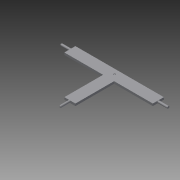
# Autodesk Inventor part: Motor_Mount
Saved by Autodesk Inventor 2015 (Build 190159000, 159)
## iProperties
Created: 2016-02-14
Part Number: Motor_Mount
Material: Generic
Document SubType Name: Modeling
Designer: david_000
Density: 1 g/cm^3
Appearance: Default
Author: david_000
Autodesk Inventor part; units mm, degrees
ref_plane "YZ Plane" through (0, 0, 0) normal (1, 0, 0) x (0, 1, 0)
ref_plane "XZ Plane" through (0, 0, 0) normal (0, 1, 0) x (-1, 0, 0)
ref_plane "XY Plane" through (0, 0, 0) normal (0, 0, 1) x (1, 0, 0)
sketch "Sketch1" plane through (0, 0, 0) normal (0, 1, 0) x (-1, 0, 0)
  line L0 (-254, 0) -> (-254, -31.75)
  line L1 (-254, -31.75) -> (0, -31.75)
  line L2 (0, -31.75) -> (0, 0)
  line L3 (-111.125, -15.875) -> (-142.875, -15.875)
  line L4 (-142.875, 0) -> (-142.875, 111.125)
  line L5 (-142.875, 111.125) -> (-111.125, 111.125)
  line L6 (-111.125, 111.125) -> (-111.125, 0)
  line L7 (0, 0) -> (-111.125, 0)
  line L8 (-142.875, 0) -> (-254, 0)
  point P0 (-127, -15.875)
  dimension "d0" = 254
  dimension "d1" = 31.75
  dimension "d5" = 15.875
  dimension "d6" = 127
  dimension "d7" = 15.875
  dimension "d8" = 127
  constraints: 18 end point, 5 parallel, 3 horizontal, 3 perpendicular
  measures "d0" distance of L1.end L0.end
  measures "d1" distance of L0.end L0.start
  measures "d5" distance of point (-127, -15.875) L3.start
  measures "d6" distance from line of L2 point (-127, -15.875)
  measures "d7" distance of point (-127, -15.875) point (-142.875, -15.875)
  measures "d8" distance of L3.end L4.end
extrude "Extrusion1" add sketch "Sketch1" along normal blind 6.35
sketch "Sketch3" plane through (0, 6.35, 0) normal (0, 1, 0) x (1, 0, 0)
  line L0 (0, 0) -> (111.125, 0) projected
  line L1 (0, 31.75) -> (0, 0) projected
  circle A0 centre (127, 17.145) radius 3.3156
  dimension "d13" = 17.145
  dimension "d14" = 127
  constraints: 1 centre point, 1 coincident
  measures "d13" distance from line of L0 point (127, 17.145)
  measures "d14" distance from line of L1 point (127, 17.145)
extrude "Extrusion3" cut sketch "Sketch3" against normal blind 1.27
sketch "Sketch4" plane through (254, 0, 0) normal (1, 0, 0) x (0, 0, -1)
  line L0 (31.75, 0) -> (0, 0) projected
  line L1 (31.75, 0) -> (31.75, 6.35) projected
  circle A0 centre (15.875, 3.175) radius 3.175
  dimension "d21" = 15.875
  dimension "d22" = 3.175
  constraints: 1 centre point, 1 coincident
  measures "d21" distance from line of L1 point (15.875, 3.175)
  measures "d22" distance from line of L0 point (15.875, 3.175)
extrude "Extrusion4" add sketch "Sketch4" along normal blind 28.575
pattern_circular "Circular Pattern2" count 3 over 180 about axis through (127, 6.35, -17.145) along (0, -1, 0) of "Extrusion4"
fillet "Fillet1" radius 3.175 1 edges at (122.555, 3.175, 138.43)
fillet "Fillet2" radius 3.175 1 edges at (-28.575, 3.175, -21.59)
body "Solid1"
